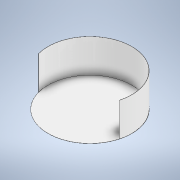
# Autodesk Inventor part: stage
Saved by Autodesk Inventor 2022 (Build 260153000, 153)
## iProperties
Created: 2021-07-12
Part Number: stage
Material: ステンレス鋼
Document SubType Name: Modeling
Designer: ken
Density: 8 g/cm^3
Appearance: 白
Author: ken
Autodesk Inventor part; units mm, degrees
ref_plane "YZ Plane" through (0, 0, 0) normal (1, 0, 0) x (0, 1, 0)
ref_plane "XZ Plane" through (0, 0, 0) normal (0, 1, 0) x (-1, 0, 0)
ref_plane "XY Plane" through (0, 0, 0) normal (0, 0, 1) x (1, 0, 0)
sketch "スケッチ1" plane through (0, 0, 0) normal (0, 1, 0) x (-1, 0, 0)
  circle A0 centre (0, -0.4884) radius 251
  point P0 (0, 0)
  dimension "d0" = 502
  constraints: 1 centre point
  measures "d0" diameter of A0
extrude "押し出し1" add sketch "スケッチ1" along normal blind 1
sketch "スケッチ2" plane through (0, 1, -0.4884) normal (0, 1, 0) x (1, 0, 0)
  circle A0 centre (0, -0.4884) radius 250
  line L0 (0, -0.4884) -> (-242.4474, -65.4519)
  line L1 (0, -0.4884) -> (251, -0.4884) construction
  line L2 (0, -0.4884) -> (242.4474, -65.4519)
  line L3 (0, -0.4884) -> (251, -0.4884) construction
  line L4 (242.4474, -65.4519) -> (-242.4474, -65.4519)
  circle A1 centre (0, -0.4884) radius 251
  point P0 (242.4474, -65.4519)
  point P1 (-242.4474, -65.4519)
  point P2 (-241.4815, -65.1931)
  point P3 (241.4815, -65.1931)
  dimension "d3" = 500
  dimension "d4" = 251
  dimension "d5" = 165
  dimension "d6" = 251
  dimension "d7" = 15
  dimension "d8" = 502
  constraints: 10 end point, 2 centre point, 2 coincident, 2 equal length, 2 horizontal
  measures "d3" diameter of A0
  measures "d4" distance of L0.start L0.end
  measures "d5" angle of L0 L1
  measures "d6" distance of L0.start L2.end
  measures "d7" angle of L2 L3
  measures "d8" diameter of A1
extrude "押し出し2" add sketch "スケッチ2" along normal blind 200 contours A0 L0 A1 L2
